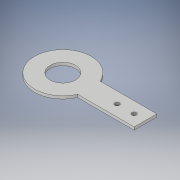
# Autodesk Inventor part: wheel tip
Saved by Autodesk Inventor 2019 (Build 230136000, 136)
## iProperties
Created: 2019-01-18
Part Number: wheel tip
Material: Generic
Document SubType Name: Modeling
Designer: s-2513225
Density: 1 g/cm^3
Appearance: Default
Author: s-2513225
Autodesk Inventor part; units mm, degrees
ref_plane "YZ Plane" through (0, 0, 0) normal (1, 0, 0) x (0, 1, 0)
ref_plane "XZ Plane" through (0, 0, 0) normal (0, 1, 0) x (-1, 0, 0)
ref_plane "XY Plane" through (0, 0, 0) normal (0, 0, 1) x (1, 0, 0)
sketch "Sketch1" plane through (0, 0, 0) normal (0, 1, 0) x (-1, 0, 0)
  line L0 (54.4994, 0) -> (79.8994, 0) construction
  arc A0 (50.8, -12.7) -> (50.8, 12.7) centre (79.8994, 0) ccw
  line L1 (0, 0) -> (19.05, 0) construction
  circle A1 centre (0, 0) radius 2.5797
  circle A2 centre (19.05, 0) radius 2.5797
  circle A3 centre (79.8994, 0) radius 14.2875
  line L2 (50.8, -12.7) -> (-12.7, -12.7)
  line L3 (50.8, 12.7) -> (-12.7, 12.7)
  line L4 (-12.7, 12.7) -> (-12.7, -12.7)
  line L5 (-12.7, 0) -> (0, 0) construction
  dimension "d6" = 19.05
  dimension "d7" = 5.1594
  dimension "d8" = 5.1594
  dimension "d9" = 28.575
  dimension "d13" = 63.5
  dimension "d14" = 63.5
  dimension "d15" = 12.7
  constraints: 12 end point, 4 centre point, 4 coincident, 3 horizontal, 2 point on circle, 1 midpoint, 1 perpendicular
  measures "d6" distance of L1.start L1.end
  measures "d7" diameter of A1
  measures "d8" diameter of A2
  measures "d9" diameter of A3
  measures "d13" distance of L2.start L2.end
  measures "d14" distance of L3.start L3.end
  measures "d15" distance of L5.start L5.end
extrude "Extrusion1" add sketch "Sketch1" along normal blind 3.175
body "Solid1"
